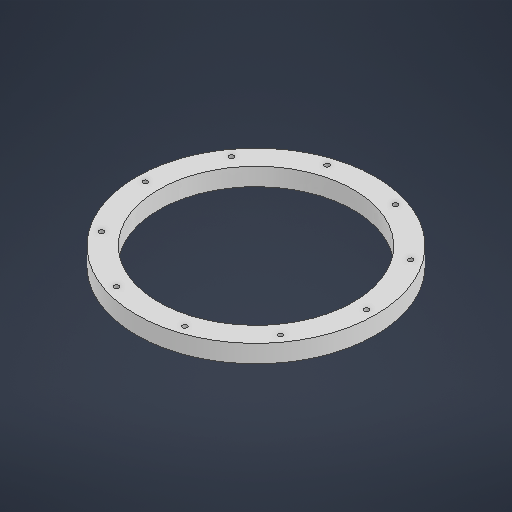
# Autodesk Inventor part: Cylinder Spacer (x3)
Saved by Autodesk Inventor 2025 (Build 290162000, 162)
## iProperties
Created: 2024-04-28
Part Number: Cylinder Spacer (x3)
Material: Generic
Document SubType Name: Modeling
Designer: Thienan Hoang
Density: 1 g/cm^3
Appearance: Default
Author: Thienan Hoang
Autodesk Inventor part; units mm, degrees
ref_plane "YZ Plane" through (0, 0, 0) normal (1, 0, 0) x (0, 1, 0)
ref_plane "XZ Plane" through (0, 0, 0) normal (0, 1, 0) x (-1, 0, 0)
ref_plane "XY Plane" through (0, 0, 0) normal (0, 0, 1) x (1, 0, 0)
sketch "Sketch1" plane through (0, 0, 0) normal (0, 1, 0) x (-1, 0, 0)
  circle A0 centre (0, 0) radius 135
  circle A1 centre (0, 0) radius 110
  dimension "d0" = 270
  dimension "d1" = 220
  constraints: 2 centre point, 2 coincident
  measures "d0" diameter of A0
  measures "d1" diameter of A1
extrude "Extrusion1" add sketch "Sketch1" along normal mid plane 20
sketch "Sketch3" plane through (0, 10, 0) normal (0, 1, 0) x (1, 0, 0)
  circle A0 centre (0, 0) radius 125
  circle A1 centre (125, 0) radius 2.5
  circle A2 centre (101.1271, 73.4732) radius 2.5
  circle A3 centre (38.6271, 118.8821) radius 2.5
  circle A4 centre (-38.6271, 118.8821) radius 2.5
  circle A5 centre (-101.1271, 73.4732) radius 2.5
  circle A6 centre (-125, 0) radius 2.5
  circle A7 centre (-101.1271, -73.4732) radius 2.5
  circle A8 centre (-38.6271, -118.8821) radius 2.5
  circle A9 centre (38.6271, -118.8821) radius 2.5
  circle A10 centre (101.1271, -73.4732) radius 2.5
  dimension "d7" = 250
  dimension "d8" = 5
  dimension "d11" = 360
  constraints: 10 centre point, 1 coincident, 1 horizontal alignment, 23 other
  measures "d8" diameter of A1
hole "Hole1" at (125, 10, 0) at (101.1271, 10, 73.4732) at (38.6271, 10, 118.8821) at (-38.6271, 10, 118.8821) at (-101.1271, 10, 73.4732) at (-125, 10, 0) at (-101.1271, 10, -73.4732) at (-38.6271, 10, -118.8821) at (38.6271, 10, -118.8821) at (101.1271, 10, -73.4732) direction (0, -1, 0) diameter 5.5 end through all
body "Solid1"
